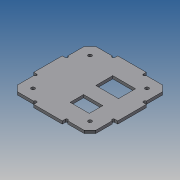
# Autodesk Inventor part: Tapa Enchufes b
Saved by Autodesk Inventor 2017 (Build 210142000, 142)
## iProperties
Part Number: Tapa Enchufes b
Material: Genérico
Document SubType Name: Modeling
Designer: Leo
Density: 1 g/cm^3
Appearance: Valor por defecto
Author: Leo
Autodesk Inventor part; units mm, degrees
ref_plane "YZ Plane" through (0, 0, 0) normal (1, 0, 0) x (0, 1, 0)
ref_plane "XZ Plane" through (0, 0, 0) normal (0, 1, 0) x (-1, 0, 0)
ref_plane "XY Plane" through (0, 0, 0) normal (0, 0, 1) x (1, 0, 0)
sketch "Boceto1" plane through (0, 0, 0) normal (0, 0, 1) x (1, 0, 0)
  line L0 (-59, 20) -> (-59, -20)
  line L1 (-59, -20) -> (-55, -20)
  arc A0 (-55, -24) -> (-55, -20) centre (-55, -22) ccw
  line L2 (-55, -24) -> (-55, -47)
  line L3 (-55, -47) -> (-47, -55)
  line L4 (-47, -55) -> (-24, -55)
  arc A1 (-20, -55) -> (-24, -55) centre (-22, -55) ccw
  line L5 (-20, -55) -> (-20, -59)
  line L6 (-20, -59) -> (20, -59)
  line L7 (20, -59) -> (20, -55)
  arc A2 (24, -55) -> (20, -55) centre (22, -55) ccw
  line L8 (24, -55) -> (47, -55)
  line L9 (47, -55) -> (55, -47)
  line L10 (27.1297, 0) -> (-27.1297, 0) construction
  line L11 (0, -24.7936) -> (0, 24.7936) construction
  arc A3 (-55, 20) -> (-55, 24) centre (-55, 22) ccw
  line L12 (-55, 24) -> (-55, 47)
  line L13 (-55, 47) -> (-47, 55)
  line L14 (-47, 55) -> (-24, 55)
  arc A4 (-24, 55) -> (-20, 55) centre (-22, 55) ccw
  line L15 (-20, 55) -> (-20, 59)
  line L16 (-20, 59) -> (20, 59)
  line L17 (20, 59) -> (20, 55)
  arc A5 (20, 55) -> (24, 55) centre (22, 55) ccw
  line L18 (24, 55) -> (47, 55)
  line L19 (47, 55) -> (55, 47)
  line L20 (-55, 20) -> (-59, 20)
  line L21 (59, 20) -> (59, -20)
  line L22 (59, -20) -> (55, -20)
  arc A6 (55, -20) -> (55, -24) centre (55, -22) ccw
  line L23 (55, -24) -> (55, -47)
  line L24 (55, 24) -> (55, 47)
  arc A7 (55, 24) -> (55, 20) centre (55, 22) ccw
  line L25 (55, 20) -> (59, 20)
  circle A8 centre (40, -40) radius 2.5
  circle A9 centre (40, 40) radius 2.5
  circle A10 centre (-40, -40) radius 2.5
  circle A11 centre (-40, 40) radius 2.5
  line L26 (32.5, 7.5) -> (32.5, 31.5)
  line L27 (32.5, 31.5) -> (0.5, 31.5)
  line L28 (0.5, 31.5) -> (0.5, 7.5)
  line L29 (0.5, 7.5) -> (32.5, 7.5)
  line L30 (-19, 35) -> (-19, 4) construction
  line L31 (-19, 4) -> (52, 4) construction
  line L32 (52, 4) -> (52, 35) construction
  line L33 (52, 35) -> (-19, 35) construction
  line L34 (30, -12) -> (3, -12)
  line L35 (3, -12) -> (3, -31)
  line L36 (3, -31) -> (30, -31)
  line L37 (30, -31) -> (30, -12)
  point P0 (0, 0)
  point P1 (0, 0)
  point P2 (-59, 0)
  point P3 (0, 59)
  point P4 (16.5, 35)
  point P5 (16.5, 31.5)
  point P6 (52, 19.5)
  point P7 (32.5, 19.5)
  point P8 (16.5, -12)
  point P9 (16.5, 7.5)
  dimension "d0" = 40
  dimension "d1" = 4
  dimension "d2" = 2
  dimension "d3" = 110
  dimension "d4" = 118
  dimension "d5" = 4
  dimension "d6" = 8
  dimension "d7" = 5
  dimension "d8" = 80
  dimension "d9" = 80
  dimension "d10" = 24
  dimension "d11" = 32
  dimension "d12" = 31
  dimension "d13" = 71
  dimension "d14" = 3
  dimension "d15" = 20
  dimension "d16" = 19
  dimension "d17" = 27
  dimension "d19" = 24
  constraints: 76 end point, 28 symmetric about line, 16 point on circle, 13 point on line, 12 centre point, 11 perpendicular, 10 midpoint, 7 parallel, 5 horizontal, 3 tangent, 2 equal radius, 2 horizontal alignment, 2 vertical, 2 vertical alignment, 1 coincident, 8 other
  measures "d0" distance of L0.start L0.end
  measures "d1" distance between parallel lines of L2 L0
  measures "d2" radius of A3
  measures "d3" distance between parallel lines of L24 L12
  measures "d4" distance between parallel lines of L6 L16
  measures "d5" distance between parallel lines of L16 L18
  measures "d6" horizontal distance of L8.end L9.end
  measures "d7" diameter of A8
  measures "d8" distance of A9.centre A8.centre
  measures "d9" distance of A10.centre A8.centre
  measures "d10" distance of L26.start L26.end
  measures "d11" distance of L26.end L27.end
  measures "d12" distance of L30.start L30.end
  measures "d13" distance of L30.end L31.end
  measures "d14" distance between parallel lines of L24 L32
  measures "d15" distance between parallel lines of L18 L33
  measures "d16" distance of L34.end L35.end
  measures "d17" distance of L34.start L34.end
  measures "d19" diameter of L34 L10
extrude "Extrusión1" add sketch "Boceto1" along normal blind 4
equation "\"d5\" = d1"
equation "\"d9\" = d8"
